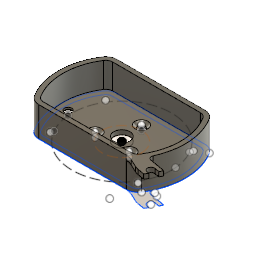
Wedge Holder v2 (Autodesk Fusion 360 design; units mm, degrees)
Autodesk Fusion 360 part; units mm, degrees
note: some values were not read from the file. Set by a fixed rule: the direction of a hole.
sketch "Sketch1" plane through (0, 0, 0) normal (0, 1, 0) x (1, 0, 0)
  circle A0 centre (0, 0) radius 8.5 construction
  circle A1 centre (0, 0) radius 3.5
  line L0 (19.0329, 17) -> (-19.0329, 17)
  line L1 (-19.0329, -17) -> (19.0329, -17)
  line L2 (-19.0329, -15) -> (19.0329, -15)
  line L3 (19.0329, 15) -> (-19.0329, 15)
  arc A2 (21.5706, -13.6) -> (21.5706, 13.6) centre (0, 0) ccw
  arc A3 (-21.5706, 13.6) -> (-21.5706, -13.6) centre (0, 0) ccw
  arc A4 (-23.2624, 14.6667) -> (-23.2624, -14.6667) centre (0, 0) ccw
  arc A5 (23.2624, -14.6667) -> (23.2624, 14.6667) centre (0, 0) ccw
  arc A6 (-19.0329, 17) -> (-23.2624, 14.6667) centre (-19.0329, 12) ccw
  arc A7 (23.2624, 14.6667) -> (19.0329, 17) centre (19.0329, 12) ccw
  arc A8 (19.0329, -17) -> (23.2624, -14.6667) centre (19.0329, -12) ccw
  arc A9 (-23.2624, -14.6667) -> (-19.0329, -17) centre (-19.0329, -12) ccw
  arc A10 (-19.0329, 15) -> (-21.5706, 13.6) centre (-19.0329, 12) ccw
  arc A11 (21.5706, 13.6) -> (19.0329, 15) centre (19.0329, 12) ccw
  arc A12 (-21.5706, -13.6) -> (-19.0329, -15) centre (-19.0329, -12) ccw
  arc A13 (19.0329, -15) -> (21.5706, -13.6) centre (19.0329, -12) ccw
  circle A14 centre (0, 0) radius 21.5 construction
  line L4 (32.8427, -14.743) -> (32.1741, -16.1502)
  line L5 (30.075, -15.763) -> (32.1741, -16.1502)
  line L6 (32.8427, -14.743) -> (26.1108, -13.5277)
  line L7 (21.7239, -17.6492) -> (25.1303, -19.2322)
  line L8 (29.7361, -20.292) -> (26.8466, -19.7746)
  line L9 (30.63, -18.9157) -> (29.6034, -18.7247)
  arc A15 (30.2243, -15.7906) -> (29.6034, -18.7247) centre (29.8779, -17.25) ccw
  arc A16 (32.1741, -16.1502) -> (32.8427, -14.743) centre (0, 0) ccw
  arc A17 (29.7361, -20.292) -> (30.63, -18.9157) centre (0, 0) ccw
  arc A18 (25.1303, -19.2322) -> (26.8466, -19.7746) centre (28.0804, -12.8842) ccw
  arc A19 (25.0129, -11.4282) -> (23.2624, 14.6667) centre (0, 0) ccw
  arc A20 (18.925, -16.9988) -> (23.2624, -14.6667) centre (19.0329, -12) ccw
  arc A21 (25.0129, -11.4282) -> (26.1108, -13.5277) centre (26.3773, -12.0516) ccw
  arc A22 (21.7239, -17.6492) -> (18.925, -16.9988) centre (18.7739, -23.9972) ccw
  dimension "d2" = 7
  dimension "d4" = 360
  dimension "d9" = 5
  dimension "d10" = 3
  dimension "d11" = 3
  dimension "d14" = 43
  dimension "d17" = 360
  dimension "d23" = 7
  dimension "d24" = 1.5
  dimension "d25" = 7
  measures "d2" diameter of A1
  measures "d9" radius of A6
  measures "d10" radius of A10
  measures "d11" radius of A12
  measures "d14" diameter of A14
  measures "d23" radius of A18
  measures "d24" radius of A21
  measures "d25" radius of A22
ref_plane "WorkPlane2" through (0, 2, 0) normal (0, 1, 0) x (-1, 0, 0)
extrude "Extrude1" add sketch "Sketch1" along normal blind 2 contours L1 A5 A8 L4 L5 L6 L7 L8 L9 A15 A17 A18 A20 A21 A22 makes body 1
extrude "Extrude2" add sketch "Sketch1" along normal blind 2 separate body contours L2 L3 A2 A3 A10 A11 A12 A13 makes body 2
extrude "Extrude3" add sketch "Sketch1" along normal blind 12.9 contours L0 L1 A4 A5 A6 A7 A8 A9 A19 A20 A22 bodies 2 1
hole "Hole1" at (-18.6195, 0, 10.75) at (-21.4182, 0, 1.8738) at (18.6195, 0, -10.75) at (21.4182, 0, -1.8738) direction (0, 1, 0) diameter 3.2 depth 2 tip angle 118 countersink diameter 5.6 countersink angle 90 bodies 2
ref_plane "WorkPlane1" through (0, 2, 0) normal (0, 1, 0) x (0, 0, 1)
sketch "Sketch2" plane through (0, 2, 0) normal (0, 1, 0) x (1, 0, 0)
hole "Hole2" at (0.0001, 2, -8.5) at (-7.3613, 2, 4.2499) at (7.3612, 2, 4.2501) direction (0, -1, 0) diameter 3.2 depth 2 tip angle 118 countersink diameter 5.6 countersink angle 90 bodies 2
extrude "Extrude4" cut sketch "Sketch1" along normal blind 2 contours L1 A5 A8 L4 L5 L6 L7 L8 L9 A15 A17 A18 A20 A21 A22 bodies 2
extrude "Extrude5" add sketch "Sketch1" against normal blind 2 from surface at 12.9 contours L1 A5 A8 L4 L5 L6 L7 L8 L9 A15 A17 A18 A20 A21 A22 bodies 2
equation "d35 = 3.2 mm + 1.2 mm + 1.2 mm"
equation "d42 = 3.2 mm + 1.2 mm + 1.2 mm"
